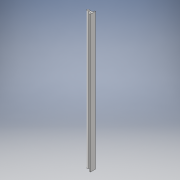
# Autodesk Inventor part: supportedLinearRail12mm_30inches
Saved by Autodesk Inventor 2018 (Build 220112000, 112)
## iProperties
Created: 2020-03-10
Part Number: supportedLinearRail12mm_30inches
Material: Generic
Document SubType Name: Modeling
Designer: natha
Density: 1 g/cm^3
Appearance: Default
Author: natha
Autodesk Inventor part; units mm, degrees
ref_plane "YZ Plane" through (0, 0, 0) normal (1, 0, 0) x (0, 1, 0)
ref_plane "XZ Plane" through (0, 0, 0) normal (0, 1, 0) x (-1, 0, 0)
ref_plane "XY Plane" through (0, 0, 0) normal (0, 0, 1) x (1, 0, 0)
sketch "Sketch1" plane through (0, 0, 0) normal (0, 1, 0) x (-1, 0, 0)
  line L0 (-6, 0) -> (0, 0) construction
  line L1 (-27, 15) -> (-27, -15)
  line L2 (-27, 15) -> (-23, 15)
  line L3 (-27, -15) -> (-23, -15)
  line L4 (-5.8057, 1.5145) -> (-23, 6)
  line L5 (-5.8057, -1.5145) -> (-23, -6)
  arc A0 (-5.8057, -1.5145) -> (-5.8057, 1.5145) centre (-0.0058, 0) ccw
  line L6 (-23, 15) -> (-23, 6)
  line L7 (-23, -6) -> (-23, -15)
  dimension "d6" = 30
  dimension "d7" = 4
  dimension "d8" = 4
  dimension "d10" = 5.9944
  constraints: 16 end point, 3 horizontal, 2 point on circle, 2 vertical, 1 centre point, 1 collinear
  measures "d6" distance of L1.start L1.end
  measures "d7" distance of L1.start L2.end
  measures "d8" distance of L1.end L3.end
  measures "d10" radius of A0
extrude "Extrusion1" add sketch "Sketch1" along normal blind 762
body "Solid1"
